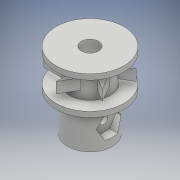
# Autodesk Inventor part: wheelSpindle
Saved by Autodesk Inventor 2018 (Build 220112000, 112)
## iProperties
Created: 2017-10-22
Part Number: wheelSpindle
Material: Generic
Document SubType Name: Modeling
Designer: Prakash
Density: 1 g/cm^3
Appearance: Default
Author: Prakash
Autodesk Inventor part; units mm, degrees
ref_plane "XZ Plane" through (0, 0, 0) normal (0, 1, 0) x (-1, 0, 0)
ref_plane "XY Plane" through (0, 0, 0) normal (0, 0, 1) x (1, 0, 0)
sketch "Sketch1" plane through (0, 0, 0) normal (0, 0, 1) x (1, 0, 0)
  circle A0 centre (0, 0) radius 7.5
  circle A1 centre (0, 0) radius 12.5
  circle A2 centre (0, 0) radius 3.175
  circle A3 centre (0, 0) radius 8.175
  dimension "d18" = 6.35
  dimension "d19" = 16.35
  dimension "d40" = 15
  dimension "d41" = 5
  constraints: 4 centre point, 4 coincident
  measures "d18" diameter of A2
  measures "d19" diameter of A3
  measures "d40" diameter of A0
  measures "d41" radial gap between concentric circles of A1 A0
extrude "Extrusion1" add sketch "Sketch1" along normal blind 14 contours A0 | A2
extrude "Extrusion2" add sketch "Sketch1" along normal blind 2 contours A1 | A3
sketch "Sketch2" plane through (0, 0, 14) normal (0, 0, 1) x (1, 0, 0)
  circle A0 centre (0, 0) radius 7.5 projected
  circle A1 centre (0, 0) radius 12.5 projected
extrude "Extrusion3" add sketch "Sketch2" against normal blind 2
ref_plane "Work Plane1" through (0, 0, 7) normal (0, 0, -1) x (-1, 0, 0)
extrude "Extrusion5" cut sketch "Sketch1" along normal up to surface (14 mm away) contours A2
extrude "Extrusion6" add sketch "Sketch1" against normal blind 14 contours A0 | A3
ref_plane "Work Plane2" through (8.175, 0, 0) normal (1, 0, 0) x (0, 1, 0)
sketch "Sketch4" plane through (8.175, 0, 0) normal (1, 0, 0) x (0, 1, 0)
  line L0 (8.175, 0) -> (-8.175, 0) projected
  line L1 (-8.175, -14) -> (8.175, -14) projected
  line L2 (0, 0) -> (0, -14)
  line L3 (-2.3094, -11) -> (-4.6188, -7)
  line L4 (-4.6188, -7) -> (-2.3094, -3)
  line L5 (-2.3094, -3) -> (2.3094, -3)
  line L6 (2.3094, -3) -> (4.6188, -7)
  line L7 (4.6188, -7) -> (2.3094, -11)
  line L8 (2.3094, -11) -> (-2.3094, -11)
  point P0 (0, -7)
  point P1 (0, -11)
  dimension "d24" = 8
  constraints: 14 end point, 3 midpoint, 1 point on line, 13 other
  measures "d24" distance between parallel lines of L4 L7
hole "Hole1" at (8.175, 0, -7) direction (-1, 0, 0) diameter 3 end up to face face through (0, 0, 0) facing (0, 0, 1) round with radius 3.175 far side yes
extrude "Extrusion7" cut sketch "Sketch4" against normal blind 3.175
sketch "Sketch8" plane through (0, 0, 7) normal (0, 0, -1) x (-1, 0, 0)
  circle A0 centre (0, 0) radius 7.5 projected
  circle A1 centre (0, 0) radius 12.5 construction
  line L0 (0, -7.5) -> (0, -12.5)
  circle A2 centre (0, 0) radius 12.5 projected
  line L1 (0, -12.5) -> (-3.3398, -6.7154)
  line L2 (0, -12.5) -> (6.6795, -12.5) construction
  line L3 (6.4952, -3.75) -> (10.8253, -6.25)
  line L4 (10.8253, -6.25) -> (4.1458, -6.25)
  line L5 (10.8253, -6.25) -> (14.1651, -0.4654) construction
  line L6 (6.4952, 3.75) -> (10.8253, 6.25)
  line L7 (10.8253, 6.25) -> (7.4855, 0.4654)
  line L8 (10.8253, 6.25) -> (7.4855, 12.0346) construction
  line L9 (0, 7.5) -> (0, 12.5)
  line L10 (0, 12.5) -> (3.3398, 6.7154)
  line L11 (0, 12.5) -> (-6.6795, 12.5) construction
  line L12 (-6.4952, 3.75) -> (-10.8253, 6.25)
  line L13 (-10.8253, 6.25) -> (-4.1458, 6.25)
  line L14 (-10.8253, 6.25) -> (-14.1651, 0.4654) construction
  line L15 (-6.4952, -3.75) -> (-10.8253, -6.25)
  line L16 (-10.8253, -6.25) -> (-7.4855, -0.4654)
  line L17 (-10.8253, -6.25) -> (-7.4855, -12.0346) construction
  circle A3 centre (0, 0) radius 7.5
  dimension "d50" = 30
  dimension "d53" = 360
  constraints: 36 end point, 2 vertical, 1 centre point, 1 coincident, 1 equal length, 1 horizontal, 1 vertical alignment, 58 other
  measures "d50" angle of L1 L0
extrude "Extrusion8" add sketch "Sketch8" along normal mid plane 4 contours A0 L6 L7 | L3 L4 A0 | A0 L9 L10 | L0 L1 A0 | L13 A0 L12 | L16 A0 L15
body "Solid1"
